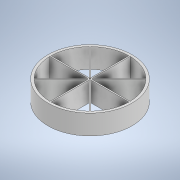
# Autodesk Inventor part: FeedWheel
Saved by Autodesk Inventor 2020 (Build 240168000, 168)
## iProperties
Created: 2020-03-05
Part Number: FeedWheel
Material: Generic
Document SubType Name: Modeling
Designer: jared.jones280
Density: 1 g/cm^3
Appearance: Default
Author: jared.jones280
Autodesk Inventor part; units mm, degrees
ref_plane "YZ Plane" through (0, 0, 0) normal (1, 0, 0) x (0, 1, 0)
ref_plane "XZ Plane" through (0, 0, 0) normal (0, 1, 0) x (-1, 0, 0)
ref_plane "XY Plane" through (0, 0, 0) normal (0, 0, 1) x (1, 0, 0)
sketch "Sketch1" plane through (0, 0, 0) normal (0, 1, 0) x (-1, 0, 0)
  circle A0 centre (0, 0) radius 50.8
  circle A1 centre (0, 0) radius 53.975
  dimension "d0" = 101.6
  dimension "d1" = 107.95
  constraints: 2 centre point, 2 coincident
  measures "d0" diameter of A0
  measures "d1" diameter of A1
extrude "Extrusion1" add sketch "Sketch1" along normal blind 25.4 contours A0 | A1
sketch "Sketch2" plane through (0, 25.4, 0) normal (0, 1, 0) x (1, 0, 0)
  circle A0 centre (0, 0) radius 50.8
  dimension "d4" = 101.6
  constraints: 1 centre point, 1 coincident
  measures "d4" diameter of A0
extrude "Extrusion2" cut sketch "Sketch2" against normal blind 22.225
sketch "Sketch3" plane through (0, 3.175, 0) normal (0, 1, 0) x (1, 0, 0)
  line L0 (-0.7937, 25.8929) -> (0.7937, -25.8929) construction
  line L1 (0.7937, 25.8929) -> (-0.7937, -25.8929) construction
  circle A0 centre (0, 0) radius 53.975 projected
  line L2 (-0.7937, 1.9214) -> (-17.916, 19.0437)
  line L3 (0.7938, 1.9213) -> (17.9468, 19.0743)
  line L4 (0.0335, 1.0941) -> (-0.0357, 1.1633)
  line L5 (0.7937, -1.9112) -> (17.9683, -19.0858)
  line L6 (0.0332, -1.0843) -> (-0.0353, -1.1529)
  line L7 (-0.7938, -1.9113) -> (-17.8495, -18.967)
  line L8 (-0.0332, -1.0842) -> (0.0353, -1.1528)
  line L9 (-0.0335, 1.094) -> (0.0357, 1.1632)
  line L10 (-25.8929, 0.7937) -> (-0.7937, 0.0243) construction
  line L11 (0, 0) -> (25.8929, -0.7937) construction
  line L12 (-25.8929, 0.7937) -> (-1.9112, 0.7937)
  line L13 (-0.0243, 0.7937) -> (0.0243, 0.7937)
  line L14 (1.9113, 0.7937) -> (25.8929, 0.7937)
  line L15 (-0.7937, 1.9214) -> (-0.7937, 25.8929)
  line L16 (-0.7937, -25.8929) -> (-0.7938, -1.9113)
  line L17 (-0.7937, -0.0243) -> (-0.7937, 0.0243)
  line L18 (-1.9213, -0.7937) -> (-25.8929, -0.7937)
  line L19 (25.8929, -0.7937) -> (1.9214, -0.7937)
  line L20 (0.0243, -0.7937) -> (-0.0243, -0.7937)
  line L21 (0.7937, -1.9112) -> (0.7937, -25.8929)
  line L22 (0.7937, 25.8929) -> (0.7938, 1.9213)
  line L23 (0.7937, 0.0243) -> (0.7937, -0.0243)
  line L24 (25.8929, 0.7937) -> (0, 0) construction
  line L25 (-0.7937, -0.0243) -> (-25.8929, -0.7937) construction
  line L26 (19.0693, 17.9518) -> (1.9113, 0.7937)
  line L27 (1.1529, 0.0353) -> (1.0843, -0.0332)
  line L28 (19.0909, -17.9632) -> (1.9214, -0.7937)
  line L29 (1.1633, -0.0357) -> (1.0941, 0.0335)
  line L30 (-18.9721, -17.8445) -> (-1.9213, -0.7937)
  line L31 (-1.1632, -0.0357) -> (-1.094, 0.0335)
  line L32 (-19.0386, 17.9211) -> (-1.9112, 0.7937)
  line L33 (-1.1528, 0.0353) -> (-1.0842, -0.0332)
  line L34 (0.7937, 25.8929) -> (0.7937, 52.3915)
  line L35 (0.7937, 52.3915) -> (-0.7937, 52.3915)
  line L36 (-0.7937, 52.3915) -> (-0.7937, 25.8929)
  line L37 (-19.0386, 17.9211) -> (-38.1124, 36.995)
  line L38 (-38.1124, 36.995) -> (-36.9899, 38.1176)
  line L39 (-36.9899, 38.1176) -> (-17.916, 19.0437)
  line L40 (-25.8929, -0.7937) -> (-52.6358, -0.7937)
  line L41 (-52.6358, -0.7937) -> (-52.6358, 0.7937)
  line L42 (-52.6358, 0.7937) -> (-25.8929, 0.7937)
  line L43 (-17.8495, -18.967) -> (-36.1442, -37.2617)
  line L44 (-36.1442, -37.2617) -> (-37.2668, -36.1392)
  line L45 (-37.2668, -36.1392) -> (-18.9721, -17.8445)
  line L46 (0.7937, -25.8929) -> (0.7937, -52.94)
  line L47 (0.7937, -52.94) -> (-0.7937, -52.94)
  line L48 (-0.7937, -52.94) -> (-0.7937, -25.8929)
  line L49 (17.9683, -19.0858) -> (36.3915, -37.509)
  line L50 (36.3915, -37.509) -> (37.5141, -36.3864)
  line L51 (37.5141, -36.3864) -> (19.0909, -17.9632)
  line L52 (25.8929, -0.7937) -> (52.8491, -0.7937)
  line L53 (52.8491, -0.7937) -> (52.8491, 0.7937)
  line L54 (52.8491, 0.7937) -> (25.8929, 0.7937)
  line L55 (19.0693, 17.9518) -> (38.1125, 36.995)
  line L56 (38.1125, 36.995) -> (36.99, 38.1176)
  line L57 (36.99, 38.1176) -> (17.9468, 19.0743)
  point P0 (0.7938, -0.7937)
  point P1 (-0.7938, 0.7937)
  point P2 (-0.7938, -0.7937)
  point P3 (0.7938, 0.7937)
  dimension "d7" = 1.5875
  dimension "d8" = 1.5875
  dimension "d9" = 1.5875
  dimension "d13" = 1.5875
  constraints: 112 end point, 58 parallel, 10 point on line, 3 horizontal, 20 other
  measures "d7" distance of L21.end L16.start
  measures "d8" distance of L14.end L11.end
  measures "d9" distance of L3.end L26.start
  measures "d13" distance of L2.end L32.start
sketch "Sketch5" plane through (0, 3.175, 0) normal (0, 1, 0) x (1, 0, 0)
  circle A0 centre (0, 0) radius 50.8 projected
  circle A1 centre (0, 0) radius 50.8 projected
  circle A2 centre (0, 0) radius 50.8 projected
  circle A3 centre (0, 0) radius 50.8 projected
  circle A4 centre (0, 0) radius 50.8 projected
  circle A5 centre (0, 0) radius 50.8 projected
  circle A6 centre (0, 0) radius 50.8 projected
  circle A7 centre (0, 0) radius 50.8 projected
extrude "Extrusion5" cut sketch "Sketch5" against normal blind 22.225
sketch "Sketch6" plane through (0, 25.4, 0) normal (0, 1, 0) x (1, 0, 0)
  line L0 (0.635, 0.635) -> (-0.635, 0.635)
  line L1 (-0.635, 0.635) -> (-0.635, -0.635)
  line L2 (-0.635, -0.635) -> (0.635, -0.635)
  line L3 (0.635, -0.635) -> (0.635, 0.635)
  line L4 (0.635, 0.635) -> (-0.635, -0.635) construction
  line L5 (-0.635, 0.635) -> (0.635, -0.635) construction
  point P0 (0, 0)
  dimension "d21" = 1.27
  dimension "d22" = 1.27
  constraints: 12 end point, 2 midpoint, 2 parallel, 1 horizontal, 1 perpendicular
  measures "d21" distance of L2.end L1.end
  measures "d22" distance of L1.end L0.end
extrude "Extrusion6" add sketch "Sketch6" along normal blind 0.635
extrude "Extrusion7" add sketch "Sketch3" along normal blind 22.225 and the other way blind 3.175 contours L15 L36 L35 L34 L22 L3 L57 L56 L55 L26 L14 L54 L53 L52 L19 L28 L51 L50 L49 L5 L21 L46 L47 L48 L16 L7 L43 L44 L45 L30 L18 L40 L41 L42 L12 L32 L37 L38 L39 L2
body "Solid1"
